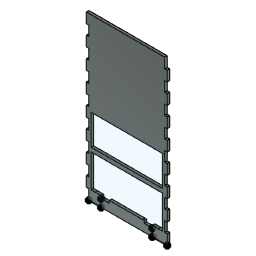
Dice Tower (Front) (Autodesk Fusion 360 design; units mm, degrees)
Autodesk Fusion 360 part; units mm, degrees
note: some values were not read from the file. Set by a fixed rule: which sketch regions a step uses.
sketch "Sketch2" plane through (0, 0, 0) normal (0, 0, 1) x (1, 0, 0)
sketch "Sketch3" plane through (0, 0, 0) normal (0, 1, 0) x (1, 0, 0)
  line L0 (85.725, 0) -> (101.6, 0)
  line L1 (88.9, -50.8) -> (85.725, -50.8)
  line L2 (187.325, -12.7) -> (184.15, -12.7)
  line L3 (104.4448, -12.7) -> (104.4448, -9.525)
  line L4 (88.9, -12.7) -> (85.725, -12.7)
  line L5 (85.725, -25.4) -> (85.725, -12.7)
  line L6 (91.7448, -12.7) -> (104.4448, -12.7)
  line L7 (88.9, -63.5) -> (88.9, -50.8)
  line L8 (181.3052, -12.7) -> (168.6052, -12.7)
  line L9 (88.9, -76.2) -> (88.9, -63.5)
  line L10 (181.3052, -53.975) -> (91.7448, -53.975)
  line L11 (85.725, 0) -> (87.3125, 0)
  line L12 (91.7448, 0) -> (91.7448, -12.7)
  line L13 (88.9, -50.8) -> (88.9, -38.1)
  line L14 (88.9, -25.4) -> (88.9, -12.7)
  line L15 (176.2252, 0) -> (181.3052, 0)
  line L16 (187.325, -38.1) -> (184.15, -38.1)
  line L17 (158.4452, -12.7) -> (156.5402, -12.7)
  line L18 (96.8248, -12.7) -> (104.4448, -12.7)
  line L19 (168.6052, -12.7) -> (176.2252, -12.7)
  line L20 (91.7448, -12.7) -> (96.8248, -12.7)
  line L21 (88.9, -38.1) -> (88.9, -25.4)
  line L22 (168.6052, -12.7) -> (168.6052, -9.525)
  line L23 (96.8248, 0) -> (91.7448, 0)
  line L24 (187.325, -25.4) -> (184.15, -25.4)
  line L25 (88.9, -25.4) -> (85.725, -25.4)
  line L26 (114.6048, -12.7) -> (156.5402, -12.7)
  line L27 (158.4452, -9.525) -> (158.4452, -12.7)
  line L28 (114.6048, -9.525) -> (114.6048, -12.7)
  line L29 (187.325, 0) -> (187.325, -12.7)
  line L30 (181.3052, -12.7) -> (176.2252, -12.7)
  line L31 (187.325, 0) -> (184.15, 0)
  line L32 (85.725, 0) -> (96.8248, 0)
  line L33 (187.325, 0) -> (176.2252, 0)
  line L34 (184.15, -12.7) -> (184.15, 0)
  line L35 (184.15, -25.4) -> (184.15, -12.7)
  line L36 (88.9, -139.7) -> (85.725, -139.7)
  line L37 (88.9, -101.6) -> (88.9, -95.25)
  line L38 (88.9, -127) -> (85.725, -127)
  line L39 (88.9, -95.25) -> (88.9, -88.9)
  line L40 (184.15, -101.6) -> (184.15, -88.9)
  line L41 (88.9, -114.3) -> (88.9, -101.6)
  line L42 (187.325, -101.6) -> (187.325, -114.3)
  line L43 (184.15, -127) -> (184.15, -114.3)
  line L44 (88.9, -127) -> (88.9, -114.3)
  line L45 (187.325, -101.6) -> (184.15, -101.6)
  line L46 (187.325, -139.7) -> (187.325, -127)
  line L47 (184.15, -139.7) -> (187.325, -139.7)
  line L48 (88.9, -114.3) -> (85.725, -114.3)
  line L49 (88.9, -139.7) -> (88.9, -127)
  line L50 (187.325, -114.3) -> (187.325, -101.6)
  line L51 (187.325, -127) -> (184.15, -127)
  line L52 (88.9, -88.9) -> (85.725, -88.9)
  line L53 (91.7448, -97.155) -> (181.3052, -97.155)
  line L54 (85.725, -101.6) -> (85.725, -88.9)
  line L55 (88.9, -101.6) -> (85.725, -101.6)
  line L56 (187.325, -127) -> (187.325, -139.7)
  line L57 (184.15, -88.9) -> (187.325, -88.9)
  line L58 (184.15, -114.3) -> (187.325, -114.3)
  line L59 (85.725, -127) -> (85.725, -114.3)
  line L60 (184.15, 0) -> (184.15, -203.2)
  line L61 (85.725, -203.2) -> (88.9, -203.2)
  line L62 (88.9, 0) -> (88.9, -203.2)
  line L63 (88.9, -165.1) -> (88.9, -152.4)
  line L64 (187.325, -152.4) -> (187.325, -165.1)
  line L65 (184.15, -203.2) -> (184.15, -190.5)
  line L66 (184.15, -152.4) -> (184.15, -139.7)
  line L67 (88.9, -203.2) -> (88.9, -190.5)
  line L68 (85.725, -152.4) -> (85.725, -139.7)
  line L69 (88.9, -165.1) -> (85.725, -165.1)
  line L70 (88.9, -190.5) -> (85.725, -190.5)
  line L71 (88.9, -177.8) -> (85.725, -177.8)
  line L72 (184.15, -177.8) -> (187.325, -177.8)
  line L73 (184.15, -190.5) -> (184.15, -177.8)
  line L74 (88.9, -152.4) -> (88.9, -139.7)
  line L75 (184.15, -165.1) -> (187.325, -165.1)
  line L76 (187.325, -177.8) -> (187.325, -190.5)
  line L77 (88.9, -152.4) -> (85.725, -152.4)
  line L78 (187.325, -152.4) -> (184.15, -152.4)
  line L79 (184.15, -190.5) -> (187.325, -190.5)
  line L80 (184.15, -76.2) -> (187.325, -76.2)
  line L81 (181.3052, 0) -> (181.3052, -12.7)
  line L82 (91.7448, -59.055) -> (181.3052, -59.055)
  line L83 (187.325, -165.1) -> (187.325, -152.4)
  line L84 (91.7448, -59.055) -> (91.7448, -97.155)
  line L85 (88.9, -63.5) -> (85.725, -63.5)
  line L86 (184.15, -177.8) -> (184.15, -165.1)
  line L87 (184.15, -50.8) -> (184.15, -38.1)
  line L88 (85.725, 0) -> (187.325, 0)
  line L89 (184.15, -63.5) -> (187.325, -63.5)
  line L90 (187.325, -25.4) -> (187.325, -38.1)
  line L91 (187.325, 0) -> (175.26, 0)
  line L92 (184.15, -76.2) -> (184.15, -63.5)
  line L93 (181.3052, -59.055) -> (181.3052, -97.155)
  line L94 (187.325, -50.8) -> (187.325, -63.5)
  line L95 (168.6052, -9.525) -> (158.4452, -9.525)
  line L96 (184.15, -38.1) -> (184.15, -25.4)
  line L97 (85.725, -76.2) -> (85.725, -63.5)
  line L98 (85.725, -177.8) -> (85.725, -165.1)
  line L99 (91.7448, -12.7) -> (91.7448, -53.975)
  line L100 (85.725, -50.8) -> (85.725, -38.1)
  line L101 (104.4448, -9.525) -> (114.6048, -9.525)
  line L102 (184.15, -50.8) -> (187.325, -50.8)
  line L103 (88.9, -177.8) -> (88.9, -165.1)
  line L104 (181.3052, -12.7) -> (181.3052, -53.975)
  line L105 (187.325, -76.2) -> (187.325, -88.9)
  line L106 (88.9, -190.5) -> (88.9, -177.8)
  line L107 (184.15, -88.9) -> (184.15, -76.2)
  line L108 (184.15, -203.2) -> (85.725, -203.2)
  line L109 (88.9, -76.2) -> (85.725, -76.2)
  line L110 (88.9, -88.9) -> (88.9, -76.2)
  line L111 (88.9, -38.1) -> (85.725, -38.1)
  line L112 (85.725, 0) -> (88.9, 0)
  line L113 (91.7448, -53.975) -> (91.7448, -59.055)
  line L114 (85.725, -203.2) -> (85.725, -190.5)
  line L115 (184.15, -63.5) -> (184.15, -50.8)
  point P0 (187.325, 0)
  dimension "d68" = 11.0998
  dimension "d69" = 11.0998
  dimension "d70" = 12.7
  dimension "d71" = 12.7
  dimension "d72" = 5.08
  dimension "d73" = 5.08
  dimension "d74" = 41.275
  dimension "d75" = 5.08
  dimension "d76" = 5.08
  dimension "d77" = 38.1
  dimension "d78" = 3.175
  dimension "d79" = 3.175
  dimension "d80" = 3.175
  dimension "d81" = 3.175
  dimension "d82" = 12.7
  dimension "d83" = 12.7
  dimension "d84" = 12.7
  dimension "d85" = 12.7
  dimension "d86" = 12.7
  dimension "d87" = 12.7
  dimension "d88" = 12.7
  dimension "d89" = 12.7
  dimension "d90" = 6.35
  dimension "d91" = 6.35
  dimension "d92" = 12.7
  dimension "d93" = 12.7
  dimension "d94" = 12.7
  dimension "d95" = 12.7
  dimension "d96" = 12.7
  dimension "d97" = 12.7
  dimension "d98" = 12.7
  dimension "d99" = 12.7
  dimension "d100" = 3.175
  dimension "d101" = 10.16
  dimension "d102" = 3.175
  dimension "d103" = 10.16
  constraint coincident P0 L29.start
  constraint perpendicular L29 L108
  constraint perpendicular L108 L114
  constraint perpendicular L29 L88
  constraint perpendicular L29 L91
  constraint perpendicular L0 L114
  constraint perpendicular L11 L114
  constraint coincident L23.start L88
  constraint perpendicular L29 L33
  constraint perpendicular L12 L23
  constraint perpendicular L81 L91
  constraint perpendicular L20 L99
  constraint perpendicular L30 L104
  constraint perpendicular L10 L113
  constraint perpendicular L82 L93
  constraint perpendicular L82 L84
  constraint perpendicular L29 L79
  constraint perpendicular L73 L79
  constraint coincident L72.end L29
  constraint perpendicular L29 L72
  constraint perpendicular L72 L86
  constraint perpendicular L29 L75
  constraint collinear L29 L76
  constraint perpendicular L75 L83
  constraint perpendicular L78 L83
  constraint parallel L31 L91
  constraint perpendicular L60 L108
  constraint perpendicular L66 L78
  constraint perpendicular L29 L47
  constraint perpendicular L46 L47
  constraint coincident L43.start L60
  constraint perpendicular L51 L60
  constraint perpendicular L43 L51
  constraint perpendicular L43 L58
  constraint perpendicular L50 L58
  constraint midpoint L40.start L60
  constraint perpendicular L45 L60
  constraint perpendicular L40 L45
  constraint parallel L60 L107
  constraint parallel L60 L92
  constraint parallel L60 L115
  constraint parallel L60 L87
  constraint parallel L87 L96
  constraint parallel L35 L60
  constraint perpendicular L29 L57
  constraint coincident L80.end L29
  constraint perpendicular L29 L80
  constraint perpendicular L29 L89
  constraint coincident L94.start L29
  constraint perpendicular L29 L102
  constraint coincident L24.start L29
  constraint collinear L29 L64
  constraint collinear L29 L56
  constraint collinear L29 L42
  constraint collinear L29 L105
  constraint collinear L29 L94
  constraint collinear L29 L90
  constraint perpendicular L61 L114
  constraint perpendicular L112 L114
  constraint perpendicular L67 L108
  constraint perpendicular L70 L114
  constraint perpendicular L70 L106
  constraint coincident L71.end L114
  constraint perpendicular L71 L114
  constraint perpendicular L71 L103
  constraint coincident L69.end L114
  constraint perpendicular L69 L114
  constraint perpendicular L63 L69
  constraint coincident L68.start L114
  constraint perpendicular L77 L114
  constraint perpendicular L74 L77
  constraint coincident L36.end L114
  constraint perpendicular L36 L114
  constraint perpendicular L36 L49
  constraint coincident L38.end L114
  constraint perpendicular L38 L114
  constraint perpendicular L38 L44
  constraint coincident L48.end L114
  constraint perpendicular L48 L114
  constraint perpendicular L41 L48
  constraint perpendicular L55 L114
  constraint perpendicular L37 L55
  constraint parallel L39 L62
  constraint coincident L52.end L114
  constraint perpendicular L52 L114
  constraint perpendicular L52 L110
  constraint coincident L97.start L114
  constraint perpendicular L109 L114
  constraint perpendicular L9 L109
  constraint coincident L85.end L114
  constraint perpendicular L85 L114
  constraint perpendicular L7 L85
  constraint coincident L1.end L114
  constraint perpendicular L1 L114
  constraint perpendicular L1 L13
  constraint coincident L100.end L114
  constraint perpendicular L111 L114
  constraint perpendicular L21 L111
  constraint perpendicular L21 L25
  constraint perpendicular L14 L25
  constraint perpendicular L4 L14
  constraint collinear L98 L114
  constraint coincident L54.start L114
  constraint collinear L68 L98
  constraint collinear L59 L68
  constraint collinear L54 L59
  constraint collinear L54 L97
  constraint collinear L97 L100
  constraint collinear L5 L100
  constraint perpendicular L8 L81
  constraint collinear L18 L19
  constraint perpendicular L6 L12
  constraint perpendicular L3 L18
  constraint perpendicular L3 L101
  constraint perpendicular L28 L101
  constraint collinear L18 L26
  constraint perpendicular L22 L95
  constraint perpendicular L27 L95
  measures "d68" distance of L0.start L23.start
  measures "d69" distance of P0 L15.start
  measures "d70" distance of L19.end L15.start
  measures "d71" distance of L23.start L18.start
  measures "d72" distance of L15.end L15.start
  measures "d73" distance of L23.start L12.start
  measures "d74" distance of L10.end L6.start
  measures "d75" distance of L10.start L82.end
  measures "d76" distance of L82.start L10.end
  measures "d77" distance of L53.start L82.start
  measures "d78" distance of L64.start L66.start
  measures "d79" distance of L31.end P0
  measures "d80" distance of L61.start L61.end
  measures "d81" distance of L0.start L62.start
  measures "d82" distance of L61.end L67.end
  measures "d83" distance of L71.start L67.end
  measures "d84" distance of L71.start L63.start
  measures "d85" distance of L63.end L63.start
  measures "d86" distance of L63.end L36.start
  measures "d87" distance of L38.start L36.start
  measures "d88" distance of L41.start L38.start
  measures "d89" distance of L37.start L41.start
  measures "d90" distance of L37.end L37.start
  measures "d91" distance of L37.end L39.end
  measures "d92" distance of L9.start L39.end
  measures "d93" distance of L9.start L7.start
  measures "d94" distance of L1.start L7.start
  measures "d95" distance of L13.end L1.start
  measures "d96" distance of L13.end L14.start
  measures "d97" distance of L4.start L14.start
  measures "d98" distance of L8.end L8.start
  measures "d99" distance of L3.start L6.start
  measures "d100" distance of L3.end L3.start
  measures "d101" distance of L28.start L3.end
  measures "d102" distance of L8.end L22.end
  measures "d103" distance of L27.start L22.end
extrude "Extrude1" add sketch "Sketch3" along normal blind 3.175 contours L0 L7 L9 L10 L12 L13 L14 L21 L32 L33 L34 L35 L37 L39 L40 L41 L43 L44 L49 L60 L62 L63 L65 L66 L67 L73 L74 L81 L86 L87 L88 L91 L92 L96 L99 L103 L104 L106 L107 L108 L110 L115 | L0 L3 L6 L8 L12 L15 L17 L18 L19 L20 L22 L23 L26 L27 L28 L30 L32 L33 L81 L88 L91 L95 L101 | L4 L5 L14 L25 L62 | L1 L13 L62 L100 L111 | L9 L62 L85 L97 L109 | L2 L29 L31 L33 L34 L60 L88 L91 | L37 L39 L52 L54 L55 L62 | L16 L24 L60 L90 L96 | L38 L44 L48 L59 L62 | L60 L89 L94 L102 L115 | L36 L62 L68 L74 L77 | L57 L60 L80 L105 L107 | L62 L69 L71 L98 L103 | L42 L45 L50 L58 L60 | L61 L62 L67 L70 L108 L114 | L46 L47 L51 L56 L60 | L60 L64 L75 L78 L83 | L60 L72 L73 L76 L79
sketch "Sketch4" plane through (0, 0, 0) normal (0, -1, 0) x (1, 0, 0)
  line L0 (168.6052, 12.7) -> (168.6052, 9.525)
  line L1 (168.6052, 9.525) -> (158.4452, 9.525)
  line L2 (158.4452, 9.525) -> (158.4452, 12.7)
  line L3 (158.4452, 12.7) -> (156.5402, 12.7)
  line L4 (156.5402, 12.7) -> (114.6048, 12.7)
  line L5 (114.6048, 12.7) -> (114.6048, 9.525)
  line L6 (114.6048, 9.525) -> (104.4448, 9.525)
  line L7 (104.4448, 9.525) -> (104.4448, 12.7)
  line L8 (104.4448, 12.7) -> (96.8248, 12.7)
  line L9 (96.8248, 12.7) -> (91.7448, 12.7)
  line L10 (91.7448, 12.7) -> (91.7448, 53.975)
  line L11 (91.7448, 53.975) -> (181.3052, 53.975)
  line L12 (181.3052, 53.975) -> (181.3052, 12.7)
  line L13 (181.3052, 12.7) -> (176.2252, 12.7)
  line L14 (176.2252, 12.7) -> (168.6052, 12.7)
  line L15 (91.7448, 59.055) -> (91.7448, 97.155)
  line L16 (91.7448, 97.155) -> (181.3052, 97.155)
  line L17 (181.3052, 97.155) -> (181.3052, 59.055)
  line L18 (181.3052, 59.055) -> (91.7448, 59.055)
  line L19 (184.15, 190.5) -> (184.15, 203.2)
  line L20 (184.15, 203.2) -> (85.725, 203.2)
  line L21 (85.725, 203.2) -> (85.725, 190.5)
  line L22 (85.725, 190.5) -> (88.9, 190.5)
  line L23 (88.9, 190.5) -> (88.9, 177.8)
  line L24 (88.9, 177.8) -> (85.725, 177.8)
  line L25 (85.725, 177.8) -> (85.725, 165.1)
  line L26 (85.725, 165.1) -> (88.9, 165.1)
  line L27 (88.9, 165.1) -> (88.9, 152.4)
  line L28 (88.9, 152.4) -> (85.725, 152.4)
  line L29 (85.725, 152.4) -> (85.725, 139.7)
  line L30 (85.725, 139.7) -> (88.9, 139.7)
  line L31 (88.9, 139.7) -> (88.9, 127)
  line L32 (88.9, 127) -> (85.725, 127)
  line L33 (85.725, 127) -> (85.725, 114.3)
  line L34 (85.725, 114.3) -> (88.9, 114.3)
  line L35 (88.9, 114.3) -> (88.9, 101.6)
  line L36 (88.9, 101.6) -> (85.725, 101.6)
  line L37 (85.725, 101.6) -> (85.725, 88.9)
  line L38 (85.725, 88.9) -> (88.9, 88.9)
  line L39 (88.9, 88.9) -> (88.9, 76.2)
  line L40 (88.9, 76.2) -> (85.725, 76.2)
  line L41 (85.725, 76.2) -> (85.725, 63.5)
  line L42 (85.725, 63.5) -> (88.9, 63.5)
  line L43 (88.9, 63.5) -> (88.9, 50.8)
  line L44 (88.9, 50.8) -> (85.725, 50.8)
  line L45 (85.725, 50.8) -> (85.725, 38.1)
  line L46 (85.725, 38.1) -> (88.9, 38.1)
  line L47 (88.9, 38.1) -> (88.9, 25.4)
  line L48 (88.9, 25.4) -> (85.725, 25.4)
  line L49 (85.725, 25.4) -> (85.725, 12.7)
  line L50 (85.725, 12.7) -> (88.9, 12.7)
  line L51 (88.9, 12.7) -> (88.9, 0)
  line L52 (88.9, 0) -> (187.325, 0)
  line L53 (187.325, 0) -> (187.325, 12.7)
  line L54 (187.325, 12.7) -> (184.15, 12.7)
  line L55 (184.15, 12.7) -> (184.15, 25.4)
  line L56 (184.15, 25.4) -> (187.325, 25.4)
  line L57 (187.325, 25.4) -> (187.325, 38.1)
  line L58 (187.325, 38.1) -> (184.15, 38.1)
  line L59 (184.15, 38.1) -> (184.15, 50.8)
  line L60 (184.15, 50.8) -> (187.325, 50.8)
  line L61 (187.325, 50.8) -> (187.325, 63.5)
  line L62 (187.325, 63.5) -> (184.15, 63.5)
  line L63 (184.15, 63.5) -> (184.15, 76.2)
  line L64 (184.15, 76.2) -> (187.325, 76.2)
  line L65 (187.325, 76.2) -> (187.325, 88.9)
  line L66 (187.325, 88.9) -> (184.15, 88.9)
  line L67 (184.15, 88.9) -> (184.15, 101.6)
  line L68 (184.15, 101.6) -> (187.325, 101.6)
  line L69 (187.325, 101.6) -> (187.325, 114.3)
  line L70 (187.325, 114.3) -> (184.15, 114.3)
  line L71 (184.15, 114.3) -> (184.15, 127)
  line L72 (184.15, 127) -> (187.325, 127)
  line L73 (187.325, 127) -> (187.325, 139.7)
  line L74 (187.325, 139.7) -> (184.15, 139.7)
  line L75 (184.15, 139.7) -> (184.15, 152.4)
  line L76 (184.15, 152.4) -> (187.325, 152.4)
  line L77 (187.325, 152.4) -> (187.325, 165.1)
  line L78 (187.325, 165.1) -> (184.15, 165.1)
  line L79 (184.15, 165.1) -> (184.15, 177.8)
  line L80 (184.15, 177.8) -> (187.325, 177.8)
  line L81 (187.325, 177.8) -> (187.325, 190.5)
  line L82 (187.325, 190.5) -> (184.15, 190.5)
  line L83 (88.9, 0) -> (104.14, 0)
  line L84 (168.6052, 9.525) -> (168.6052, 0)
  line L85 (168.6052, 0) -> (187.325, 0)
  line L86 (104.4448, 9.525) -> (104.4448, 0)
  constraint coincident L51.end L52.start
  constraint coincident L52 L83.end
  constraint perpendicular L51 L83
  constraint coincident L0.end L1.start
  constraint coincident L52 L84.end
  constraint perpendicular L1 L84
  constraint coincident L52.end L53.start
  constraint coincident L6.end L7.start
  constraint coincident L52 L86.end
  constraint perpendicular L52 L86
equation "d68 = 0.5 in - 0.063 in"
equation "d74 = 1.5 in + 0.125 in"
